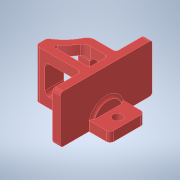
# Autodesk Inventor part: Stopper
Saved by Autodesk Inventor 2021 (Build 250183000, 183)
## iProperties
Created: 2020-03-04
Part Number: Stopper
Material: Polypropylen
Document SubType Name: Modeling
Designer: kaebi
Density: 0.899 g/cm^3
Appearance: Glatt - Rot
Description: Stopper
Stock Number: FOB 031 A
Mass: 4.75057 g
Surface Area: 42.1268 cm^2
Volume: 5.28428 cm^3
Author: kaebi
Autodesk Inventor part; units mm, degrees
ref_plane "YZ Plane" through (0, 0, 0) normal (1, 0, 0) x (0, 1, 0)
ref_plane "XZ Plane" through (0, 0, 0) normal (0, 1, 0) x (-1, 0, 0)
ref_plane "XY Plane" through (0, 0, 0) normal (0, 0, 1) x (1, 0, 0)
sketch "Skizze1" plane through (0, 0, 0) normal (0, 1, 0) x (-1, 0, 0)
  line L0 (33.5, -9) -> (4.5, -9)
  line L1 (4.5, -9) -> (2.5, -10)
  line L2 (2.5, -10) -> (-5.5, -10)
  line L3 (-5.5, -10) -> (-5.5, 10)
  line L4 (-5.5, 10) -> (2.5, 10)
  line L5 (2.5, 10) -> (4.5, 9)
  line L6 (4.5, 9) -> (33.5, 9)
  line L7 (33.5, 9) -> (33.5, -9)
  circle A0 centre (0, 0) radius 2.75 construction
  line L8 (81.8, 0) -> (-20.05, 0) projected
  line L9 (4.5, -9) -> (-5.5, -9)
  line L10 (4.5, 9) -> (-5.5, 9)
  circle A1 centre (44.5, -17) radius 22.75
  point P0 (23.202993, -9)
  point P1 (33.5, 2.913877)
  dimension "d0" = 5.5
  dimension "d1" = 5.5
  dimension "d2" = 20
  dimension "d3" = 8
  dimension "d4" = 2
  dimension "d5" = 18
  dimension "d6" = 39
  dimension "d57" = 45.5
  dimension "d58" = 8
  dimension "d59" = 11
  constraints: 20 end point, 5 perpendicular, 2 centre point, 2 equal length, 2 parallel, 2 point on line, 1 coincident, 1 horizontal, 2 other
  measures "d0" distance from line of A0.centre L3
  measures "d1" diameter of A0
  measures "d2" distance of L2.end L3.end
  measures "d3" distance of L1.end L2.end
  measures "d4" horizontal distance of L0.end L1.end
  measures "d5" distance of L6.end L0.start
  measures "d6" distance between parallel lines of L7 L3
  measures "d57" diameter of A1
  measures "d58" distance from line of L0 A1.centre
  measures "d59" distance from line of L7 A1.centre
extrude "Extrusion1" add sketch "Skizze1" along normal mid plane 5 contours L0 L9 L3 L8 A1 | L8 L3 L10 L6 L7 A1
sketch "Skizze4" plane through (0, 2.5, 0) normal (0, 1, 0) x (1, 0, 0)
  line L0 (5.5, -9) -> (5.5, 9) projected
  point P0 (0, 0)
  point P1 (0.5, 0)
  dimension "d81" = 5
  constraints: 1 horizontal alignment
  measures "d81" distance from line of L0 point (0.5, 0)
hole "Bohrung1" at (0.5, 2.5, 0) direction (0, -1, 0) diameter 5 end through all
fillet "Rundung1" radius 2 4 edges at (-33.5, 0, 9) (5.5, 0, 9) (5.5, 0, -9) (-33.5, 0, 2.9139)
sketch "Skizze5" plane through (0, 2.5, 0) normal (0, 1, 0) x (1, 0, 0)
  line L0 (-33.5, -4.060924) -> (-33.5, -7)
  arc A0 (-33.5, -7) -> (-31.5, -9) centre (-31.5, -7) ccw
  line L1 (-31.5, -9) -> (3.5, -9)
  line L2 (5.5, -7) -> (5.5, 7)
  line L3 (3.5, 9) -> (-23.202993, 9)
  circle A1 centre (0.5, 0) radius 2.5
  line L4 (-31.5, -9) -> (3.5, -9)
  line L5 (-5.5, -9) -> (-5.5, 9)
  line L6 (3.5, 9) -> (-23.202993, 9)
  arc A2 (5.5, 7) -> (3.5, 9) centre (3.5, 7) ccw
  arc A3 (3.5, -9) -> (5.5, -7) centre (3.5, -7) ccw
  arc A4 (-32.550505, -2.359031) -> (-23.202993, 9) centre (-44.5, 17) ccw
  arc A5 (-32.550505, -2.359031) -> (-33.5, -4.060924) centre (-31.5, -4.060924) ccw
  point P0 (0, 0)
  point P1 (-22.45789, 9)
  point P2 (-4.736068, -9)
  point P3 (-4.736068, 9)
  point P4 (-21.721317, 9)
  dimension "d27" = 11
  constraints: 2 end point, 2 point on line, 1 perpendicular
  measures "d27" distance between parallel lines of L2 L5
extrude "Extrusion2" add sketch "Skizze5" along normal blind 20 contours A5 A4 L3 L5 L1 A0 L0
sketch "Skizze6" plane through (0, 22.5, 0) normal (0, 1, 0) x (1, 0, 0)
  line L0 (-31.5, -9) -> (-5.5, -9)
  line L1 (-5.5, -9) -> (-5.5, 9)
  line L2 (-5.5, 9) -> (-23.202993, 9)
  line L3 (-33.5, -4.060924) -> (-33.5, -7)
  arc A0 (-33.5, -7) -> (-31.5, -9) centre (-31.5, -7) ccw
  line L4 (-9.5, -5) -> (-30.179997, -5)
  arc A1 (-30.179997, -5) -> (-21.153426, 5) centre (-44.5, 17) ccw
  line L5 (-21.153426, 5) -> (-9.5, 5)
  line L6 (-9.5, 5) -> (-9.5, -5)
  arc A2 (-32.550505, -2.359031) -> (-23.202993, 9) centre (-44.5, 17) ccw
  arc A3 (-32.550505, -2.359031) -> (-33.5, -4.060924) centre (-31.5, -4.060924) ccw
  arc A4 (-32.550505, -2.359031) -> (-23.202993, 9) centre (-44.5, 17) ccw
  point P0 (0, 0)
  point P1 (-22.646735, 8.378947)
  dimension "d28" = 4
  dimension "d77" = 4
  dimension "d78" = 26.25
  constraints: 6 end point, 2 point on circle, 1 centre point, 1 concentric, 1 other
  measures "d28" distance between parallel lines of L0 L4
  measures "d77" distance between parallel lines of L2 L5
  measures "d78" radius of A1
extrude "Extrusion3" cut sketch "Skizze6" against normal up to surface (25 mm away) contours L4 A1 L5 L6
fillet "Rundung2" radius 1 1 edges at (-30.18, 10, 5)
sketch "Skizze7" plane through (-31.5, -2.5, 9) normal (0, 0, 1) x (1, 0, 0)
  line L0 (3, 20) -> (22, 20)
  line L1 (22, 20) -> (22, 5)
  line L2 (22, 5) -> (3, 5)
  line L3 (3, 5) -> (3, 20)
  line L4 (0, 25) -> (26, 25)
  line L5 (-2, 25) -> (-2, 0)
  line L6 (35, 0) -> (0, 0)
  line L7 (19.635074, 20) -> (22.378676, 20)
  line L8 (22.378676, 5) -> (19.635074, 5)
  line L9 (22, 25) -> (22, 0)
  point P0 (31.5, 2.5)
  point P1 (47, 0)
  dimension "d35" = 5
  dimension "d49" = 5
  dimension "d50" = 5
  constraints: 12 end point, 3 parallel, 2 horizontal, 2 point on line, 1 collinear, 1 perpendicular
  measures "d35" distance between parallel lines of L6 L2
  measures "d49" distance between parallel lines of L5 L3
  measures "d50" distance between parallel lines of L4 L0
extrude "Extrusion5" cut sketch "Skizze7" against normal up to surface (18 mm away)
sketch "Skizze9" plane through (-31.5, -2.5, 9) normal (0, 0, 1) x (1, 0, 0)
  line L0 (8.297007, 0) -> (35, 0)
  line L1 (0, 25) -> (26, 25)
  line L2 (35, 0) -> (0, 0)
  line L3 (22, 25) -> (26, 25)
  line L4 (26, 25) -> (26, 0)
  line L5 (26, 0) -> (22, 0)
  line L6 (22, 0) -> (22, 25)
  line L7 (26, 5) -> (26, 25)
  line L8 (22, 20) -> (22, 5)
  point P0 (20.54211, 0)
  point P1 (22, 0)
  point P2 (-1, 0)
  point P3 (9.978683, 0)
  constraints: 8 end point, 2 collinear, 2 parallel, 2 point on line, 1 horizontal, 1 perpendicular
extrude "Extrusion7" add sketch "Skizze9" along normal blind 15 and the other way blind 33
fillet "Rundung5" radius 1.5 16 edges at (-9.5, 0, -9) (-9.5, 20, -9) (-9.5, 20, 9) (-9.5, 0, 9) (-7.5, -2.5, -24) (-7.5, -2.5, 24) (-7.5, 22.5, 24) (-7.5, 22.5, -24) (-9.5, 20, -5) (-9.5, 20, 5) (-9.5, 17.5, 7) (-9.5, 17.5, -7) (-9.5, 2.5, -7) (-9.5, 0, -5) (-9.5, 0, 5) (-9.5, 2.5, 7)
sketch "Skizze11" plane through (-5.5, 2.5, 9) normal (1, 0, 0) x (0, 0, -1)
  circle A0 centre (9, -2.5) radius 7.5
  dimension "d51" = 15
  constraints: 1 centre point, 1 coincident
  measures "d51" diameter of A0
extrude "Extrusion8" add sketch "Skizze11" along normal blind 1
sketch "Skizze12" plane through (-5.5, 2.5, 9) normal (-1, 0, 0) x (0, 0, 1)
  line L0 (-16.071068, -5) -> (-1.928932, -5)
  arc A0 (-16.071068, -5) -> (-1.928932, -5) centre (-9, -2.5) ccw
extrude "Extrusion9" add sketch "Skizze12" along normal up to surface (4 mm away)
fillet "Rundung6" radius 2 1 edges at (-5.5, 7.5, 0)
sketch "Skizze13" plane through (-9.5, 22.5, -3.5) normal (-1, 0, 0) x (0, 0, 1)
  line L0 (-18.5, -2) -> (-12.5, -2)
  line L1 (-12.5, -2) -> (-12.5, -23)
  line L2 (-12.5, -23) -> (-18.5, -23)
  line L3 (-18.5, -23) -> (-18.5, -2)
  line L4 (19.5, -2) -> (25.5, -2)
  line L5 (25.5, -2) -> (25.5, -23)
  line L6 (25.5, -23) -> (19.5, -23)
  line L7 (19.5, -23) -> (19.5, -2)
  line L8 (-20.5, -23.5) -> (-20.5, -1.5) projected
  line L9 (-19, 0) -> (-7, 0) projected
  line L10 (-7, -25) -> (-19, -25) projected
  line L11 (14, -6.5) -> (14, 0) projected
  line L12 (27.5, -1.5) -> (27.5, -23.5) projected
  point P0 (3.5, -22.5)
  dimension "d60" = 6
  dimension "d61" = 2
  dimension "d62" = 2
  dimension "d63" = 2
  dimension "d65" = 6
  dimension "d80" = 2
  constraints: 16 end point, 4 parallel, 2 horizontal, 2 perpendicular, 2 point on line
  measures "d60" distance between parallel lines of L3 L1
  measures "d61" distance between parallel lines of L8 L3
  measures "d62" distance between parallel lines of L9 L0
  measures "d63" distance between parallel lines of L10 L2
  measures "d65" distance between parallel lines of L7 L5
  measures "d80" distance between parallel lines of L12 L5
extrude "Extrusion10" cut sketch "Skizze13" against normal blind 0.3
sketch "Skizze14" plane through (-29.8, 2.5, 2.947722) normal (0, 1, 0) x (1, 0, 0)
  line L0 (18.8, 11.947722) -> (18.8, 7.947722)
  line L1 (6.597007, 11.947722) -> (18.8, 11.947722)
  arc A0 (1.3, 3.774828) -> (6.597007, 11.947722) centre (-14.7, 19.947722) ccw
  line L2 (1.3, -6.052278) -> (1.3, 3.774828)
  arc A1 (2.028287, -0.281636) -> (8.646574, 7.947722) centre (-14.7, 19.947722) ccw
  line L3 (18.8, 7.947722) -> (8.646574, 7.947722)
  line L4 (18.8, -2.052278) -> (18.8, -6.052278)
  line L5 (2.665555, -2.052278) -> (18.8, -2.052278)
  arc A2 (2.028287, -0.281636) -> (2.665555, -2.052278) centre (2.665555, -1.052278) ccw
  line L6 (18.8, -6.052278) -> (1.3, -6.052278)
  line L7 (24.3, 11.947722) -> (18.8, 11.947722)
  line L8 (10.8, 11.947722) -> (10.8, 7.947722)
  line L9 (18.8, 7.947722) -> (8.646574, 7.947722)
  line L10 (10.8, 7.947722) -> (4.627765, 7.947722)
  arc A3 (-2.750505, 0.588691) -> (6.597007, 11.947722) centre (-14.7, 19.947722) ccw
  point P0 (29.8, 2.947722)
  point P1 (8.078683, 11.947722)
  point P2 (7.153265, 11.326669)
  point P3 (10.049165, 7.947722)
  point P4 (4.627765, 7.947722)
  point P5 (10.8, 7.947722)
  point P6 (10.8, 11.947722)
  point P7 (4.332164, 8.205011)
  point P8 (8.646574, 7.947722)
  point P9 (4.927765, 7.947722)
  point P10 (9.549165, 7.947722)
  point P11 (8.078683, 11.947722)
  dimension "d79" = 8
  constraints: 4 end point, 2 perpendicular, 2 point on line, 1 point on circle
  measures "d79" distance between parallel lines of L0 L8
extrude "Extrusion11" add sketch "Skizze14" along normal up to surface (15 mm away) contours L8 L3 L10 A0 L1
fillet "Rundung7" radius 4 1 edges at (-23.203, 10, -9)
fillet "Rundung8" radius 4 2 edges at (-21.1534, 20, -5) (-21.1534, 0, -5)
fillet "Rundung9" radius 2 6 edges at (-28.5, 2.5, 4.0864) (-22.0861, 2.5, -5) (-19, 2.5, -7) (-22.0861, 17.5, -5) (-19, 17.5, -7) (-28.5, 17.5, 4.0864)
